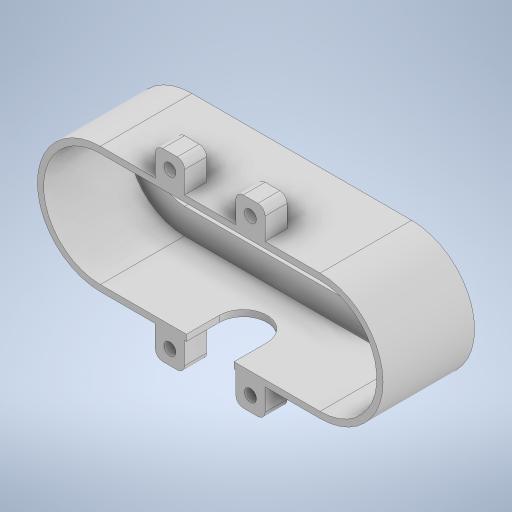
# Autodesk Inventor part: suporteBright2k
Saved by Autodesk Inventor 2023 (Build 270158000, 158)
## iProperties
Created: 2024-02-20
Part Number: suporteBright2k
Material: Generic
Document SubType Name: Modeling
Designer: brvn
Density: 1 g/cm^3
Appearance: Default
Author: brvn
Autodesk Inventor part; units mm, degrees
ref_plane "YZ Plane" through (0, 0, 0) normal (1, 0, 0) x (0, 1, 0)
ref_plane "XZ Plane" through (0, 0, 0) normal (0, 1, 0) x (-1, 0, 0)
ref_plane "XY Plane" through (0, 0, 0) normal (0, 0, 1) x (1, 0, 0)
sketch "Sketch1" plane through (0, 0, 0) normal (0, 0, 1) x (1, 0, 0)
  line L0 (-30, 0) -> (30, 0)
  line L1 (-30, -17.2) -> (30, -17.2)
  line L2 (30, 17.2) -> (-30, 17.2)
  arc A0 (-30, 17.2) -> (-30, -17.2) centre (-30, 0) ccw
  arc A1 (30, -17.2) -> (30, 17.2) centre (30, 0) ccw
  line L3 (-30, 8.5) -> (30, 8.5)
  arc A2 (30, -8.5) -> (30, 8.5) centre (30, 0) ccw
  line L4 (30, -8.5) -> (-30, -8.5)
  arc A3 (-30, 8.5) -> (-30, -8.5) centre (-30, 0) ccw
  line L5 (-47.2, 0) -> (47.2, 0)
  line L6 (0, 17.2) -> (0, -17.2)
  line L7 (-30, 15.5) -> (30, 15.5)
  arc A4 (30, -15.5) -> (30, 15.5) centre (30, 0) ccw
  line L8 (30, -15.5) -> (-30, -15.5)
  arc A5 (-30, 15.5) -> (-30, -15.5) centre (-30, 0) ccw
  point P0 (0, 0)
  point P1 (45.5, 0)
  point P2 (-45.5, 0)
  dimension "d6" = 1.7
  dimension "d12" = 31
  dimension "d13" = 91
  dimension "d14" = 7
  constraints: 20 end point, 16 point on circle, 6 centre point, 4 tangent, 3 midpoint, 3 parallel, 1 horizontal, 6 other
  measures "d6" distance between parallel lines of L2 L7
  measures "d12" distance between parallel lines of L8 L7
  measures "d13" distance of point (45.5, 0) point (-45.5, 0)
  measures "d14" distance between parallel lines of L7 L3
extrude "Extrusion1" add sketch "Sketch1" along normal blind 25 contours A5 L8 L6 L1 A0 L5 | L5 A0 L2 L6 L7 A5 | L6 L2 A1 L5 A4 L7 | L8 A4 L5 A1 L1 L6
extrude "Extrusion2" add sketch "Sketch1" along normal blind 2 contours L5 A5 L7 L6 L3 A3 | A3 L4 L6 L8 A5 L5 | L6 L7 A4 L5 A2 L3 | L4 A2 L5 A4 L8 L6
sketch "Sketch2" plane through (-30, -17.2, 25) normal (0, -1, 0) x (1, 0, 0)
  line L0 (60, -25) -> (60, 0) projected
  line L1 (0, 0) -> (60, 0) projected
  line L2 (0, -25) -> (0, 0) projected
  line L3 (30, 0) -> (30, -23) construction
  line L4 (0, -12.5) -> (60, -12.5) construction
  circle A0 centre (30, -9) radius 6.5
  line L5 (0, -2.5) -> (60, -2.5) construction
  line L6 (23.5, -9) -> (23.5, 0)
  line L7 (36.5, -9) -> (36.5, 0)
  line L8 (0, -25) -> (60, -25) projected
  point P0 (30, -25)
  dimension "d15" = 13
  dimension "d17" = 2.5
  constraints: 10 end point, 5 point on line, 3 midpoint, 3 perpendicular, 2 point on circle, 2 tangent, 1 centre point
  measures "d15" diameter of A0
  measures "d17" distance between parallel lines of L1 L5
extrude "Extrusion3" cut sketch "Sketch2" against normal up to surface (1.7 mm away) contours L7 A0 L6 L1 | A0
sketch "Sketch4" plane through (0, 0, 25) normal (0, 0, 1) x (1, 0, 0)
  line L0 (-6.5, -17.2) -> (-6.5, -15.5) projected
  line L1 (-6.5, -15.5) -> (-30, -15.5) projected
  arc A0 (-30, 15.5) -> (-30, -15.5) centre (-30, 0) ccw projected
  line L2 (-30, 15.5) -> (30, 15.5) projected
  arc A1 (30, -15.5) -> (30, 15.5) centre (30, 0) ccw projected
  line L3 (30, -15.5) -> (6.5, -15.5) projected
  line L4 (6.5, -15.5) -> (6.5, -17.2) projected
  line L5 (6.5, -17.2) -> (30, -17.2) projected
  arc A2 (30, -17.2) -> (30, 17.2) centre (30, 0) ccw projected
  line L6 (30, 17.2) -> (-30, 17.2) projected
  arc A3 (-30, 17.2) -> (-30, -17.2) centre (-30, 0) ccw projected
  line L7 (-30, -17.2) -> (-6.5, -17.2) projected
  line L8 (-15, 17.2) -> (-7, 17.2)
  line L9 (-7, 17.2) -> (-7, 25.2)
  line L10 (-7, 25.2) -> (-15, 25.2)
  line L11 (-15, 25.2) -> (-15, 17.2)
  line L12 (-15, -17.2) -> (-7, -17.2)
  line L13 (-7, -17.2) -> (-7, -25.2)
  line L14 (-7, -25.2) -> (-15, -25.2)
  line L15 (-15, -25.2) -> (-15, -17.2)
  line L16 (7, -17.2) -> (15, -17.2)
  line L17 (15, -17.2) -> (15, -25.2)
  line L18 (15, -25.2) -> (7, -25.2)
  line L19 (7, -25.2) -> (7, -17.2)
  line L20 (7, 17.2) -> (15, 17.2)
  line L21 (15, 17.2) -> (15, 25.2)
  line L22 (15, 25.2) -> (7, 25.2)
  line L23 (7, 25.2) -> (7, 17.2)
  line L24 (0, 0) -> (0, 30) construction
  line L25 (0, 0) -> (0, -30) construction
  circle A4 centre (-11, 21.2) radius 1.65
  circle A5 centre (11, 21.2) radius 1.65
  circle A6 centre (11, -21.2) radius 1.65
  circle A7 centre (-11, -21.2) radius 1.65
  dimension "d20" = 8
  dimension "d21" = 8
  dimension "d22" = 8
  dimension "d23" = 8
  dimension "d24" = 8
  dimension "d25" = 8
  dimension "d26" = 8
  dimension "d27" = 8
  dimension "d30" = 30
  dimension "d31" = 7
  dimension "d32" = 7
  dimension "d33" = 30
  dimension "d34" = 7
  dimension "d35" = 3.3
  dimension "d36" = 3.3
  dimension "d37" = 3.3
  dimension "d38" = 3.3
  dimension "d39" = 4
  dimension "d40" = 4
  dimension "d41" = 4
  dimension "d42" = 4
  dimension "d43" = 4
  dimension "d44" = 4
  dimension "d45" = 4
  dimension "d46" = 4
  dimension "d47" = 42.4
  dimension "d48" = 22
  constraints: 36 end point, 8 parallel, 5 point on line, 4 centre point, 4 horizontal, 4 perpendicular, 2 vertical
  measures "d20" distance of L10.end L9.end
  measures "d21" distance of L9.end L8.end
  measures "d22" distance of L13.end L14.end
  measures "d23" distance of L12.end L13.end
  measures "d24" distance of L17.end L18.end
  measures "d25" distance of L16.end L17.end
  measures "d26" distance of L22.end L21.end
  measures "d27" distance of L21.end L20.end
  measures "d30" distance of L24.start L24.end
  measures "d31" distance between parallel lines of L24 L9
  measures "d32" distance between parallel lines of L24 L23
  measures "d33" distance of L24.start L25.end
  measures "d34" distance between parallel lines of L25 L19
  measures "d35" diameter of A4
  measures "d36" diameter of A5
  measures "d37" diameter of A6
  measures "d38" diameter of A7
  measures "d39" distance from line of L9 A4.centre
  measures "d40" distance from line of L10 A4.centre
  measures "d41" distance from line of L22 A5.centre
  measures "d42" distance from line of L21 A5.centre
  measures "d43" distance from line of L5 A6.centre
  measures "d44" distance from line of L17 A6.centre
  measures "d45" distance from line of L14 A7.centre
  measures "d46" distance from line of L13 A7.centre
  measures "d47" distance of A7.centre A4.centre
  measures "d48" distance of A5.centre A4.centre
extrude "Extrusion4" add sketch "Sketch4" against normal blind 6 contours L13 L14 L15 L7 | L11 L10 L9 L6 | L23 L22 L21 L6 | L5 L17 L18 L19
sketch "Sketch5" plane through (0, 0, 19) normal (0, 0, -1) x (-1, 0, 0)
  line L0 (-7, 17.2) -> (-7, 25.2) projected
  line L1 (-7, 25.2) -> (-15, 25.2) projected
  line L2 (-15, 25.2) -> (-15, 17.2) projected
  line L3 (-7, 17.2) -> (-15, 17.2) projected
  circle A0 centre (-11, 21.2) radius 1.65 projected
  line L4 (15, 17.2) -> (15, 25.2) projected
  line L5 (15, 25.2) -> (7, 25.2) projected
  line L6 (7, 25.2) -> (7, 17.2) projected
  line L7 (15, 17.2) -> (7, 17.2) projected
  circle A1 centre (11, 21.2) radius 1.65 projected
  line L8 (-15, -17.2) -> (-15, -25.2) projected
  line L9 (-15, -25.2) -> (-7, -25.2) projected
  line L10 (-7, -25.2) -> (-7, -17.2) projected
  line L11 (-15, -17.2) -> (-7, -17.2) projected
  circle A2 centre (-11, -21.2) radius 1.65 projected
  line L12 (7, -17.2) -> (7, -25.2) projected
  line L13 (7, -25.2) -> (15, -25.2) projected
  line L14 (15, -25.2) -> (15, -17.2) projected
  line L15 (7, -17.2) -> (15, -17.2) projected
  circle A3 centre (11, -21.2) radius 1.65 projected
  circle A4 centre (-11, 21.2) radius 1.65 projected
  line L16 (-11, 24.4909) -> (-8.15, 22.8454)
  line L17 (-8.15, 22.8454) -> (-8.15, 19.5546)
  line L18 (-8.15, 19.5546) -> (-11, 17.9091)
  line L19 (-11, 17.9091) -> (-13.85, 19.5546)
  line L20 (-13.85, 19.5546) -> (-13.85, 22.8454)
  line L21 (-13.85, 22.8454) -> (-11, 24.4909)
  line L22 (11, 24.4909) -> (13.85, 22.8454)
  line L23 (13.85, 22.8454) -> (13.85, 19.5546)
  line L24 (13.85, 19.5546) -> (11, 17.9091)
  line L25 (11, 17.9091) -> (8.15, 19.5546)
  line L26 (8.15, 19.5546) -> (8.15, 22.8454)
  line L27 (8.15, 22.8454) -> (11, 24.4909)
  line L28 (-11, -24.4909) -> (-13.85, -22.8454)
  line L29 (-13.85, -22.8454) -> (-13.85, -19.5546)
  line L30 (-13.85, -19.5546) -> (-11, -17.9091)
  line L31 (-11, -17.9091) -> (-8.15, -19.5546)
  line L32 (-8.15, -19.5546) -> (-8.15, -22.8454)
  line L33 (-8.15, -22.8454) -> (-11, -24.4909)
  line L34 (11, -24.4909) -> (8.15, -22.8454)
  line L35 (8.15, -22.8454) -> (8.15, -19.5546)
  line L36 (8.15, -19.5546) -> (11, -17.9091)
  line L37 (11, -17.9091) -> (13.85, -19.5546)
  line L38 (13.85, -19.5546) -> (13.85, -22.8454)
  line L39 (13.85, -22.8454) -> (11, -24.4909)
  point P0 (0, 0)
  dimension "d51" = 5.7
  dimension "d52" = 5.7
  dimension "d53" = 5.7
  dimension "d54" = 5.7
  dimension "d55" = 30
  dimension "d56" = 30
  dimension "d57" = 30
  dimension "d58" = 30
  constraints: 48 end point, 4 coincident, 52 other
  measures "d51" distance between parallel lines of L32 L29
  measures "d52" distance between parallel lines of L38 L35
  measures "d53" distance between parallel lines of L17 L20
  measures "d54" distance between parallel lines of L23 L26
  measures "d55" angle of L1 L16
  measures "d56" angle of L5 L22
  measures "d57" angle of L13 L34
  measures "d58" angle of L9 L33
extrude "Extrusion5" cut sketch "Sketch5" against normal blind 2.5 contours A0 | L16 L17 L18 L19 L20 L21 | L22 L23 L24 L25 L26 L27 | L28 L29 L30 L31 L32 L33 | L34 L35 L36 L37 L38 L39
sketch "Sketch6" plane through (0, 0, 2) normal (0, 0, 1) x (1, 0, 0)
  line L0 (30, -15.5) -> (-30, -15.5) projected
  arc A0 (30, -15.5) -> (30, 15.5) centre (30, 0) ccw projected
  line L1 (-30, 15.5) -> (30, 15.5) projected
  arc A1 (-30, 15.5) -> (-30, -15.5) centre (-30, 0) ccw projected
  arc A2 (-30, 8.5) -> (-30, -8.5) centre (-30, 0) ccw projected
  line L2 (-30, 8.5) -> (30, 8.5) projected
  arc A3 (30, -8.5) -> (30, 8.5) centre (30, 0) ccw projected
  line L3 (30, -8.5) -> (-30, -8.5) projected
  line L4 (-7.2935, 13.5053) -> (-8.0592, 10.4573)
  line L5 (-8.0592, 10.4573) -> (-8.5137, 10.4573)
  line L6 (-8.5137, 10.4573) -> (-9.1337, 12.9866)
  line L7 (-9.1337, 12.9866) -> (-9.7363, 10.4573)
  line L8 (-9.7363, 10.4573) -> (-10.1859, 10.4573)
  line L9 (-10.1859, 10.4573) -> (-10.9639, 13.5053)
  line L10 (-10.9639, 13.5053) -> (-10.5465, 13.5053)
  line L11 (-10.5465, 13.5053) -> (-9.9339, 10.9785)
  line L12 (-9.9339, 10.9785) -> (-9.3263, 13.5053)
  line L13 (-9.3263, 13.5053) -> (-8.9138, 13.5053)
  line L14 (-8.9138, 13.5053) -> (-8.3013, 10.9488)
  line L15 (-8.3013, 10.9488) -> (-7.6912, 13.5053)
  line L16 (-7.6912, 13.5053) -> (-7.2935, 13.5053)
  line L17 (-6.9304, 10.4573) -> (-6.9304, 13.5053)
  line L18 (-6.9304, 13.5053) -> (-5.0236, 13.5053)
  line L19 (-5.0236, 13.5053) -> (-5.0236, 13.1447)
  line L20 (-5.0236, 13.1447) -> (-6.5253, 13.1447)
  line L21 (-6.5253, 13.1447) -> (-6.5253, 12.3098)
  line L22 (-6.5253, 12.3098) -> (-5.1248, 12.3098)
  line L23 (-5.1248, 12.3098) -> (-5.1248, 11.9492)
  line L24 (-5.1248, 11.9492) -> (-6.5253, 11.9492)
  line L25 (-6.5253, 11.9492) -> (-6.5253, 10.8179)
  line L26 (-6.5253, 10.8179) -> (-5.0236, 10.8179)
  line L27 (-5.0236, 10.8179) -> (-5.0236, 10.4573)
  line L28 (-5.0236, 10.4573) -> (-6.9304, 10.4573)
  spline S0 degree 2 poles (-2.5115, 11.3934) (-2.5115, 11.1662) (-2.6844, 10.8179) (-2.8277, 10.7043) knots 0 0 0 1 2 2 2
  spline S1 degree 2 poles (-2.8277, 10.7043) (-3.0006, 10.5709) (-3.3933, 10.4573) (-3.7046, 10.4573) knots 0 0 0 1 2 2 2
  line L29 (-3.7046, 10.4573) -> (-4.579, 10.4573)
  line L30 (-4.579, 10.4573) -> (-4.579, 13.5053)
  line L31 (-4.579, 13.5053) -> (-3.7713, 13.5053)
  spline S2 degree 2 poles (-3.7713, 13.5053) (-3.4452, 13.5053) (-3.1192, 13.4633) (-2.971, 13.3818) knots 0 0 0 1 2 2 2
  spline S3 degree 2 poles (-2.971, 13.3818) (-2.8055, 13.2953) (-2.6548, 13.0113) (-2.6548, 12.8186) knots 0 0 0 1 2 2 2
  spline S4 degree 2 poles (-2.6548, 12.8186) (-2.6548, 12.6037) (-2.882, 12.2629) (-3.0821, 12.1665) knots 0 0 0 1 2 2 2
  line L32 (-3.0821, 12.1665) -> (-3.0821, 12.1517)
  spline S5 degree 2 poles (-3.0821, 12.1517) (-2.8104, 12.0776) (-2.5115, 11.6849) (-2.5115, 11.3934) knots 0 0 0 1 2 2 2
  spline S6 degree 2 poles (-2.9339, 11.3761) (-2.9339, 11.549) (-3.0327, 11.7713) (-3.1809, 11.8504) knots 0 0 0 1 2 2 2
  spline S7 degree 2 poles (-3.1809, 11.8504) (-3.2773, 11.8998) (-3.5045, 11.9294) (-3.7144, 11.9294) knots 0 0 0 1 2 2 2
  line L33 (-3.7144, 11.9294) -> (-4.1739, 11.9294)
  line L34 (-4.1739, 11.9294) -> (-4.1739, 10.8031)
  line L35 (-4.1739, 10.8031) -> (-3.8454, 10.8031)
  spline S8 degree 2 poles (-3.8454, 10.8031) (-3.5786, 10.8031) (-3.2723, 10.8525) (-3.1538, 10.9315) knots 0 0 0 1 2 2 2
  spline S9 degree 2 poles (-3.1538, 10.9315) (-3.0401, 11.013) (-2.9339, 11.2156) (-2.9339, 11.3761) knots 0 0 0 1 2 2 2
  spline S10 degree 2 poles (-3.0772, 12.7618) (-3.0772, 12.8705) (-3.1513, 13.0335) (-3.2328, 13.0804) knots 0 0 0 1 2 2 2
  spline S11 degree 2 poles (-3.2328, 13.0804) (-3.3316, 13.1348) (-3.5712, 13.1595) (-3.7861, 13.1595) knots 0 0 0 1 2 2 2
  line L36 (-3.7861, 13.1595) -> (-4.1739, 13.1595)
  line L37 (-4.1739, 13.1595) -> (-4.1739, 12.2678)
  line L38 (-4.1739, 12.2678) -> (-3.7144, 12.2678)
  spline S12 degree 2 poles (-3.7144, 12.2678) (-3.5243, 12.2678) (-3.3439, 12.3073) (-3.2476, 12.3691) knots 0 0 0 1 2 2 2
  spline S13 degree 2 poles (-3.2476, 12.3691) (-3.1538, 12.4284) (-3.0772, 12.6186) (-3.0772, 12.7618) knots 0 0 0 1 2 2 2
  spline S14 degree 2 poles (-0.9184, 10.403) (-1.2148, 10.403) (-1.7162, 10.603) (-1.899, 10.8031) knots 0 0 0 1 2 2 2
  spline S15 degree 2 poles (-1.899, 10.8031) (-2.0818, 11.0007) (-2.2818, 11.5935) (-2.2818, 11.9788) knots 0 0 0 1 2 2 2
  spline S16 degree 2 poles (-2.2818, 11.9788) (-2.2818, 12.3617) (-2.0867, 12.9298) (-1.9015, 13.1397) knots 0 0 0 1 2 2 2
  spline S17 degree 2 poles (-1.9015, 13.1397) (-1.7187, 13.3447) (-1.2197, 13.5596) (-0.911, 13.5596) knots 0 0 0 1 2 2 2
  spline S18 degree 2 poles (-0.911, 13.5596) (-0.7578, 13.5596) (-0.4886, 13.5152) (-0.375, 13.4806) knots 0 0 0 1 2 2 2
  spline S19 degree 2 poles (-0.375, 13.4806) (-0.2762, 13.4485) (-0.0712, 13.3571) (0.0301, 13.3027) knots 0 0 0 1 2 2 2
  line L39 (0.0301, 13.3027) -> (0.0301, 12.8137)
  line L40 (0.0301, 12.8137) -> (-0.002, 12.8137)
  spline S20 degree 2 poles (-0.002, 12.8137) (-0.0564, 12.8631) (-0.2243, 13.0014) (-0.3453, 13.0681) knots 0 0 0 1 2 2 2
  spline S21 degree 2 poles (-0.3453, 13.0681) (-0.4614, 13.1323) (-0.7356, 13.2138) (-0.9134, 13.2138) knots 0 0 0 1 2 2 2
  spline S22 degree 2 poles (-0.9134, 13.2138) (-1.1086, 13.2138) (-1.4568, 13.0533) (-1.5878, 12.9001) knots 0 0 0 1 2 2 2
  spline S23 degree 2 poles (-1.5878, 12.9001) (-1.7162, 12.7445) (-1.8595, 12.2728) (-1.8595, 11.9788) knots 0 0 0 1 2 2 2
  spline S24 degree 2 poles (-1.8595, 11.9788) (-1.8595, 11.6651) (-1.7088, 11.2131) (-1.5779, 11.0575) knots 0 0 0 1 2 2 2
  spline S25 degree 2 poles (-1.5779, 11.0575) (-1.4494, 10.9068) (-1.1061, 10.7537) (-0.9134, 10.7537) knots 0 0 0 1 2 2 2
  spline S26 degree 2 poles (-0.9134, 10.7537) (-0.7381, 10.7537) (-0.4392, 10.8401) (-0.3231, 10.9044) knots 0 0 0 1 2 2 2
  spline S27 degree 2 poles (-0.3231, 10.9044) (-0.212, 10.9686) (-0.0465, 11.102) (0.0005, 11.1489) knots 0 0 0 1 2 2 2
  line L41 (0.0005, 11.1489) -> (0.0301, 11.1489)
  line L42 (0.0301, 11.1489) -> (0.0301, 10.6648)
  spline S28 degree 2 poles (0.0301, 10.6648) (-0.0712, 10.6178) (-0.249, 10.5314) (-0.375, 10.4919) knots 0 0 0 1 2 2 2
  spline S29 degree 2 poles (-0.375, 10.4919) (-0.5084, 10.4474) (-0.7356, 10.403) (-0.9184, 10.403) knots 0 0 0 1 2 2 2
  line L43 (0.0795, 10.4573) -> (1.107, 13.5053)
  line L44 (1.107, 13.5053) -> (1.606, 13.5053)
  line L45 (1.606, 13.5053) -> (2.6335, 10.4573)
  line L46 (2.6335, 10.4573) -> (2.2062, 10.4573)
  line L47 (2.2062, 10.4573) -> (1.9295, 11.3094)
  line L48 (1.9295, 11.3094) -> (0.7662, 11.3094)
  line L49 (0.7662, 11.3094) -> (0.4895, 10.4573)
  line L50 (0.4895, 10.4573) -> (0.0795, 10.4573)
  line L51 (1.8184, 11.6552) -> (1.3466, 13.0903)
  line L52 (1.3466, 13.0903) -> (0.8773, 11.6552)
  line L53 (0.8773, 11.6552) -> (1.8184, 11.6552)
  line L54 (5.5358, 10.4573) -> (5.1307, 10.4573)
  line L55 (5.1307, 10.4573) -> (5.1307, 13.0829)
  line L56 (5.1307, 13.0829) -> (4.3353, 11.2971)
  line L57 (4.3353, 11.2971) -> (4.0883, 11.2971)
  line L58 (4.0883, 11.2971) -> (3.3004, 13.0829)
  line L59 (3.3004, 13.0829) -> (3.3004, 10.4573)
  line L60 (3.3004, 10.4573) -> (2.9225, 10.4573)
  line L61 (2.9225, 10.4573) -> (2.9225, 13.5053)
  line L62 (2.9225, 13.5053) -> (3.4758, 13.5053)
  line L63 (3.4758, 13.5053) -> (4.2365, 11.8084)
  line L64 (4.2365, 11.8084) -> (4.9726, 13.5053)
  line L65 (4.9726, 13.5053) -> (5.5358, 13.5053)
  line L66 (5.5358, 13.5053) -> (5.5358, 10.4573)
  spline S30 degree 2 poles (9.5298, 11.3934) (9.5298, 11.1662) (9.3569, 10.8179) (9.2136, 10.7043) knots 0 0 0 1 2 2 2
  spline S31 degree 2 poles (9.2136, 10.7043) (9.0407, 10.5709) (8.648, 10.4573) (8.3368, 10.4573) knots 0 0 0 1 2 2 2
  line L67 (8.3368, 10.4573) -> (7.4624, 10.4573)
  line L68 (7.4624, 10.4573) -> (7.4624, 13.5053)
  line L69 (7.4624, 13.5053) -> (8.2701, 13.5053)
  spline S32 degree 2 poles (8.2701, 13.5053) (8.5961, 13.5053) (8.9222, 13.4633) (9.0704, 13.3818) knots 0 0 0 1 2 2 2
  spline S33 degree 2 poles (9.0704, 13.3818) (9.2359, 13.2953) (9.3865, 13.0113) (9.3865, 12.8186) knots 0 0 0 1 2 2 2
  spline S34 degree 2 poles (9.3865, 12.8186) (9.3865, 12.6037) (9.1593, 12.2629) (8.9592, 12.1665) knots 0 0 0 1 2 2 2
  line L70 (8.9592, 12.1665) -> (8.9592, 12.1517)
  spline S35 degree 2 poles (8.9592, 12.1517) (9.2309, 12.0776) (9.5298, 11.6849) (9.5298, 11.3934) knots 0 0 0 1 2 2 2
  spline S36 degree 2 poles (9.1074, 11.3761) (9.1074, 11.549) (9.0086, 11.7713) (8.8604, 11.8504) knots 0 0 0 1 2 2 2
  spline S37 degree 2 poles (8.8604, 11.8504) (8.7641, 11.8998) (8.5368, 11.9294) (8.3269, 11.9294) knots 0 0 0 1 2 2 2
  line L71 (8.3269, 11.9294) -> (7.8675, 11.9294)
  line L72 (7.8675, 11.9294) -> (7.8675, 10.8031)
  line L73 (7.8675, 10.8031) -> (8.196, 10.8031)
  spline S38 degree 2 poles (8.196, 10.8031) (8.4627, 10.8031) (8.769, 10.8525) (8.8876, 10.9315) knots 0 0 0 1 2 2 2
  spline S39 degree 2 poles (8.8876, 10.9315) (9.0012, 11.013) (9.1074, 11.2156) (9.1074, 11.3761) knots 0 0 0 1 2 2 2
  spline S40 degree 2 poles (8.9641, 12.7618) (8.9641, 12.8705) (8.89, 13.0335) (8.8085, 13.0804) knots 0 0 0 1 2 2 2
  spline S41 degree 2 poles (8.8085, 13.0804) (8.7097, 13.1348) (8.4701, 13.1595) (8.2553, 13.1595) knots 0 0 0 1 2 2 2
  line L74 (8.2553, 13.1595) -> (7.8675, 13.1595)
  line L75 (7.8675, 13.1595) -> (7.8675, 12.2678)
  line L76 (7.8675, 12.2678) -> (8.3269, 12.2678)
  spline S42 degree 2 poles (8.3269, 12.2678) (8.5171, 12.2678) (8.6974, 12.3073) (8.7937, 12.3691) knots 0 0 0 1 2 2 2
  spline S43 degree 2 poles (8.7937, 12.3691) (8.8876, 12.4284) (8.9641, 12.6186) (8.9641, 12.7618) knots 0 0 0 1 2 2 2
  line L77 (12.2913, 10.4573) -> (11.7651, 10.4573)
  line L78 (11.7651, 10.4573) -> (10.8018, 11.6701)
  line L79 (10.8018, 11.6701) -> (10.3375, 11.6701)
  line L80 (10.3375, 11.6701) -> (10.3375, 10.4573)
  line L81 (10.3375, 10.4573) -> (9.9324, 10.4573)
  line L82 (9.9324, 10.4573) -> (9.9324, 13.5053)
  line L83 (9.9324, 13.5053) -> (10.7179, 13.5053)
  spline S44 degree 2 poles (10.7179, 13.5053) (10.9797, 13.5053) (11.3329, 13.4485) (11.4934, 13.3447) knots 0 0 0 1 2 2 2
  spline S45 degree 2 poles (11.4934, 13.3447) (11.654, 13.241) (11.8392, 12.9174) (11.8392, 12.6778) knots 0 0 0 1 2 2 2
  spline S46 degree 2 poles (11.8392, 12.6778) (11.8392, 12.3444) (11.4984, 11.8924) (11.2069, 11.7837) knots 0 0 0 1 2 2 2
  line L84 (11.2069, 11.7837) -> (12.2913, 10.4573)
  spline S47 degree 2 poles (11.4169, 12.6457) (11.4169, 12.7791) (11.323, 12.9841) (11.2242, 13.0508) knots 0 0 0 1 2 2 2
  spline S48 degree 2 poles (11.2242, 13.0508) (11.1378, 13.1076) (10.9081, 13.1545) (10.7401, 13.1545) knots 0 0 0 1 2 2 2
  line L85 (10.7401, 13.1545) -> (10.3375, 13.1545)
  line L86 (10.3375, 13.1545) -> (10.3375, 12.0085)
  line L87 (10.3375, 12.0085) -> (10.6932, 12.0085)
  spline S49 degree 2 poles (10.6932, 12.0085) (10.8685, 12.0085) (11.1476, 12.0702) (11.244, 12.1665) knots 0 0 0 1 2 2 2
  spline S50 degree 2 poles (11.244, 12.1665) (11.3329, 12.2505) (11.4169, 12.4876) (11.4169, 12.6457) knots 0 0 0 1 2 2 2
  line L88 (13.5954, 10.4573) -> (12.4148, 10.4573)
  line L89 (12.4148, 10.4573) -> (12.4148, 10.7685)
  line L90 (12.4148, 10.7685) -> (12.8026, 10.7685)
  line L91 (12.8026, 10.7685) -> (12.8026, 13.1941)
  line L92 (12.8026, 13.1941) -> (12.4148, 13.1941)
  line L93 (12.4148, 13.1941) -> (12.4148, 13.5053)
  line L94 (12.4148, 13.5053) -> (13.5954, 13.5053)
  line L95 (13.5954, 13.5053) -> (13.5954, 13.1941)
  line L96 (13.5954, 13.1941) -> (13.2076, 13.1941)
  line L97 (13.2076, 13.1941) -> (13.2076, 10.7685)
  line L98 (13.2076, 10.7685) -> (13.5954, 10.7685)
  line L99 (13.5954, 10.7685) -> (13.5954, 10.4573)
  spline S51 degree 2 poles (15.3738, 10.398) (15.0503, 10.398) (14.5143, 10.5956) (14.3216, 10.7957) knots 0 0 0 1 2 2 2
  spline S52 degree 2 poles (14.3216, 10.7957) (14.129, 10.9982) (13.9239, 11.596) (13.9239, 11.9838) knots 0 0 0 1 2 2 2
  spline S53 degree 2 poles (13.9239, 11.9838) (13.9239, 12.3518) (14.1314, 12.9347) (14.3241, 13.1422) knots 0 0 0 1 2 2 2
  spline S54 degree 2 poles (14.3241, 13.1422) (14.5093, 13.3423) (15.0527, 13.5596) (15.3763, 13.5596) knots 0 0 0 1 2 2 2
  spline S55 degree 2 poles (15.3763, 13.5596) (15.5319, 13.5596) (15.8135, 13.5152) (15.9419, 13.4757) knots 0 0 0 1 2 2 2
  spline S56 degree 2 poles (15.9419, 13.4757) (16.0457, 13.446) (16.2976, 13.3373) (16.3742, 13.2978) knots 0 0 0 1 2 2 2
  line L100 (16.3742, 13.2978) -> (16.3742, 12.8087)
  line L101 (16.3742, 12.8087) -> (16.3396, 12.8087)
  spline S57 degree 2 poles (16.3396, 12.8087) (16.263, 12.8754) (16.1025, 12.9965) (15.9543, 13.0656) knots 0 0 0 1 2 2 2
  spline S58 degree 2 poles (15.9543, 13.0656) (15.8308, 13.1274) (15.5122, 13.2089) (15.3294, 13.2089) knots 0 0 0 1 2 2 2
  spline S59 degree 2 poles (15.3294, 13.2089) (14.8897, 13.2089) (14.3463, 12.5469) (14.3463, 11.9961) knots 0 0 0 1 2 2 2
  spline S60 degree 2 poles (14.3463, 11.9961) (14.3463, 11.6898) (14.4896, 11.2304) (14.6254, 11.0723) knots 0 0 0 1 2 2 2
  spline S61 degree 2 poles (14.6254, 11.0723) (14.7563, 10.9142) (15.1268, 10.7488) (15.359, 10.7488) knots 0 0 0 1 2 2 2
  spline S62 degree 2 poles (15.359, 10.7488) (15.5295, 10.7488) (15.8703, 10.7982) (15.9864, 10.8476) knots 0 0 0 1 2 2 2
  line L102 (15.9864, 10.8476) -> (15.9864, 11.6355)
  line L103 (15.9864, 11.6355) -> (15.28, 11.6355)
  line L104 (15.28, 11.6355) -> (15.28, 11.9912)
  line L105 (15.28, 11.9912) -> (16.3865, 11.9912)
  line L106 (16.3865, 11.9912) -> (16.3865, 10.6598)
  spline S63 degree 2 poles (16.3865, 10.6598) (16.31, 10.6253) (16.0482, 10.519) (15.937, 10.4869) knots 0 0 0 1 2 2 2
  spline S64 degree 2 poles (15.937, 10.4869) (15.7863, 10.4425) (15.5443, 10.398) (15.3738, 10.398) knots 0 0 0 1 2 2 2
  line L107 (19.1085, 10.4573) -> (18.7034, 10.4573)
  line L108 (18.7034, 10.4573) -> (18.7034, 11.9492)
  line L109 (18.7034, 11.9492) -> (17.3005, 11.9492)
  line L110 (17.3005, 11.9492) -> (17.3005, 10.4573)
  line L111 (17.3005, 10.4573) -> (16.8954, 10.4573)
  line L112 (16.8954, 10.4573) -> (16.8954, 13.5053)
  line L113 (16.8954, 13.5053) -> (17.3005, 13.5053)
  line L114 (17.3005, 13.5053) -> (17.3005, 12.3098)
  line L115 (17.3005, 12.3098) -> (18.7034, 12.3098)
  line L116 (18.7034, 12.3098) -> (18.7034, 13.5053)
  line L117 (18.7034, 13.5053) -> (19.1085, 13.5053)
  line L118 (19.1085, 13.5053) -> (19.1085, 10.4573)
  line L119 (20.4374, 10.4573) -> (20.4374, 13.1447)
  line L120 (20.4374, 13.1447) -> (19.4148, 13.1447)
  line L121 (19.4148, 13.1447) -> (19.4148, 13.5053)
  line L122 (19.4148, 13.5053) -> (21.865, 13.5053)
  line L123 (21.865, 13.5053) -> (21.865, 13.1447)
  line L124 (21.865, 13.1447) -> (20.8425, 13.1447)
  line L125 (20.8425, 13.1447) -> (20.8425, 10.4573)
  line L126 (20.8425, 10.4573) -> (20.4374, 10.4573)
  line L127 (25.2761, 10.4573) -> (23.3965, 10.4573)
  line L128 (23.3965, 10.4573) -> (23.3965, 10.8895)
  spline S65 degree 2 poles (23.3965, 10.8895) (23.599, 11.0797) (23.9596, 11.4329) (24.1325, 11.6231) knots 0 0 0 1 2 2 2
  spline S66 degree 2 poles (24.1325, 11.6231) (24.4808, 12.006) (24.7352, 12.4654) (24.7352, 12.7099) knots 0 0 0 1 2 2 2
  spline S67 degree 2 poles (24.7352, 12.7099) (24.7352, 12.8384) (24.6562, 13.031) (24.5845, 13.0928) knots 0 0 0 1 2 2 2
  spline S68 degree 2 poles (24.5845, 13.0928) (24.5129, 13.1545) (24.3252, 13.2163) (24.2116, 13.2163) knots 0 0 0 1 2 2 2
  spline S69 degree 2 poles (24.2116, 13.2163) (24.1029, 13.2163) (23.8806, 13.162) (23.7793, 13.12) knots 0 0 0 1 2 2 2
  spline S70 degree 2 poles (23.7793, 13.12) (23.6929, 13.0854) (23.5323, 12.9866) (23.4829, 12.952) knots 0 0 0 1 2 2 2
  line L129 (23.4829, 12.952) -> (23.4607, 12.952)
  line L130 (23.4607, 12.952) -> (23.4607, 13.3867)
  spline S71 degree 2 poles (23.4607, 13.3867) (23.5866, 13.4485) (24.0387, 13.5695) (24.2412, 13.5695) knots 0 0 0 1 2 2 2
  spline S72 degree 2 poles (24.2412, 13.5695) (24.6685, 13.5695) (25.1502, 13.1175) (25.1502, 12.7322) knots 0 0 0 1 2 2 2
  spline S73 degree 2 poles (25.1502, 12.7322) (25.1502, 12.5519) (25.0662, 12.2505) (24.9921, 12.1221) knots 0 0 0 1 2 2 2
  spline S74 degree 2 poles (24.9921, 12.1221) (24.918, 11.9887) (24.7031, 11.7269) (24.5845, 11.6009) knots 0 0 0 1 2 2 2
  spline S75 degree 2 poles (24.5845, 11.6009) (24.3919, 11.391) (23.9201, 10.9414) (23.7793, 10.8105) knots 0 0 0 1 2 2 2
  line L131 (23.7793, 10.8105) -> (25.2761, 10.8105)
  line L132 (25.2761, 10.8105) -> (25.2761, 10.4573)
  line L133 (27.9932, 10.4573) -> (27.467, 10.4573)
  line L134 (27.467, 10.4573) -> (26.3531, 11.8751)
  line L135 (26.3531, 11.8751) -> (26.1752, 11.675)
  line L136 (26.1752, 11.675) -> (26.1752, 10.4573)
  line L137 (26.1752, 10.4573) -> (25.7701, 10.4573)
  line L138 (25.7701, 10.4573) -> (25.7701, 13.5053)
  line L139 (25.7701, 13.5053) -> (26.1752, 13.5053)
  line L140 (26.1752, 13.5053) -> (26.1752, 12.1048)
  line L141 (26.1752, 12.1048) -> (27.4251, 13.5053)
  line L142 (27.4251, 13.5053) -> (27.9191, 13.5053)
  line L143 (27.9191, 13.5053) -> (26.6569, 12.1443)
  line L144 (26.6569, 12.1443) -> (27.9932, 10.4573)
  point P0 (0, 0)
  point P1 (8.4541, 11.9838)
  constraints: 1 other
extrude "Extrusion6" cut sketch "Sketch6" against normal blind 1 contours L4 L5 L6 L7 L8 L9 L10 L11 L12 L13 L14 L15 L16 | L17 L18 L19 L20 L21 L22 L23 L24 L25 L26 L27 L28 | S0 S1 L29 L30 L31 S2 S3 S4 L32 S5 | S14 S15 S16 S17 S18 S19 L39 L40 S20 S21 S22 S23 S24 S25 S26 S27 L41 L42 S28 S29 | L43 L44 L45 L46 L47 L48 L49 L50 | L54 L55 L56 L57 L58 L59 L60 L61 L62 L63 L64 L65 L66 | S30 S31 L67 L68 L69 S32 S33 S34 L70 S35 | L77 L78 L79 L80 L81 L82 L83 S44 S45 S46 L84 | L88 L89 L90 L91 L92 L93 L94 L95 L96 L97 L98 L99 | S51 S52 S53 S54 S55 S56 L100 L101 S57 S58 S59 S60 S61 S62 L102 L103 L104 L105 L106 S63 S64 | L107 L108 L109 L110 L111 L112 L113 L114 L115 L116 L117 L118 | L119 L120 L121 L122 L123 L124 L125 L126 | L127 L128 S65 S66 S67 S68 S69 S70 L129 L130 S71 S72 S73 S74 S75 L131 L132 | L133 L134 L135 L136 L137 L138 L139 L140 L141 L142 L143 L144
fillet "Fillet2" radius 2 8 edges at (-15, 25.2, 22) (15, 25.2, 22) (7, 25.2, 22) (-7, 25.2, 22) (-15, -25.2, 22) (-7, -25.2, 22) (15, -25.2, 22) (7, -25.2, 22)
equation "\"d32\" = d31"
equation "\"d33\" = d30"
equation "\"d34\" = d32"
equation "\"d36\" = d35"
equation "\"d37\" = d36"
equation "\"d38\" = d37"
equation "\"d40\" = d39"
equation "\"d41\" = d39"
equation "\"d42\" = d41"
equation "\"d43\" = d42"
equation "\"d44\" = d43"
equation "\"d45\" = d43"
equation "\"d46\" = d45"
equation "\"d51\" = d53"
equation "\"d52\" = d51"
equation "\"d54\" = d53"
equation "\"d56\" = d55"
equation "\"d58\" = d57"
body "Solid1"
